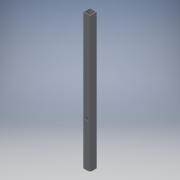
# Autodesk Inventor part: AP 2
Saved by Autodesk Inventor 2016 (Build 200138000, 138)
## iProperties
Created: 2016-02-17
Part Number: AP 2
Material: Generic
Document SubType Name: Modeling
Designer: Admin
Density: 1 g/cm^3
Appearance: Default
Author: Admin
Autodesk Inventor part; units mm, degrees
ref_plane "YZ Plane" through (0, 0, 0) normal (1, 0, 0) x (0, 1, 0)
ref_plane "XZ Plane" through (0, 0, 0) normal (0, 1, 0) x (-1, 0, 0)
ref_plane "XY Plane" through (0, 0, 0) normal (0, 0, 1) x (1, 0, 0)
sketch "Sketch1" plane through (0, 0, 0) normal (0, 1, 0) x (-1, 0, 0)
  line L0 (0, 0) -> (25.4, 0)
  line L1 (25.4, 0) -> (25.4, -25.4)
  line L2 (25.4, -25.4) -> (0, -25.4)
  line L3 (0, -25.4) -> (0, 0)
  line L4 (23.8125, -23.8125) -> (23.8125, -1.5875)
  line L5 (23.8125, -1.5875) -> (1.5875, -1.5875)
  line L6 (1.5875, -1.5875) -> (1.5875, -23.8125)
  line L7 (1.5875, -23.8125) -> (23.8125, -23.8125)
  dimension "d0" = 25.4
  dimension "d1" = 25.4
  dimension "d2" = 1.5875
  constraints: 16 end point, 4 parallel, 2 perpendicular, 1 horizontal, 3 other
  measures "d0" distance of L1.end L2.end
  measures "d1" distance of L0.end L1.end
  measures "d2" distance between parallel lines of L1 L4
extrude "Extrusion1" add sketch "Sketch1" along normal blind 508
sketch "Sketch3" plane through (-25.4, 0, 0) normal (0, 0, 1) x (1, 0, 0)
  point P0 (25.4, 0)
sketch "Sketch4" plane through (-25.4, 0, 0) normal (0, 0, 1) x (1, 0, 0)
  circle A0 centre (12.7, 168.402) radius 6.35
  line L0 (25.4, 0) -> (0, 0) projected
  dimension "d8" = 12.7
  dimension "d9" = 168.402
  constraints: 1 centre point
  measures "d8" diameter of A0
  measures "d9" distance from line of L0 A0.centre
extrude "Extrusion3" cut sketch "Sketch4" against normal blind 25.4
sketch "Sketch5" plane through (-25.4, 0, 0) normal (0, 0, 1) x (1, 0, 0)
  circle A0 centre (12.7, 168.656) radius 6.35
  line L0 (25.4, 0) -> (0, 0) projected
  dimension "d12" = 12.7
  dimension "d15" = 168.656
  constraints: 1 centre point
  measures "d12" diameter of A0
  measures "d15" distance from line of L0 A0.centre
extrude "Extrusion4" cut sketch "Sketch5" against normal blind 25.4
sketch "Sketch6" plane through (0, 0, -25.4) normal (0, 0, -1) x (-1, 0, 0)
  circle A0 centre (10.1854, 83.82) radius 6.35
  line L0 (25.4, 0) -> (0, 0) projected
  line L1 (0, 0) -> (0, 508) projected
  dimension "d16" = 12.7
  dimension "d17" = 83.82
  dimension "d18" = 10.1854
  constraints: 1 centre point
  measures "d16" diameter of A0
  measures "d17" distance from line of L0 A0.centre
  measures "d18" distance from line of L1 A0.centre
extrude "Extrusion5" cut sketch "Sketch6" against normal blind 25.4
sketch "Sketch7" plane through (0, 0, 0) normal (0, -1, 0) x (1, 0, 0)
  line L0 (0, 0) -> (-25.4, 0)
  line L1 (-25.4, 0) -> (-25.4, -25.4)
  line L2 (-25.4, -25.4) -> (0, -25.4)
  line L3 (0, -25.4) -> (0, 0)
  line L4 (-1.5875, -23.8125) -> (-23.8125, -23.8125) projected
  line L5 (-23.8125, -1.5875) -> (-1.5875, -1.5875) projected
  line L6 (-23.8125, -23.8125) -> (-1.5875, -23.8125)
  line L7 (-1.5875, -23.8125) -> (-1.5875, -1.5875)
  line L8 (-1.5875, -1.5875) -> (-23.8125, -1.5875)
  line L9 (-23.8125, -1.5875) -> (-23.8125, -23.8125)
  constraints: 16 end point, 4 parallel, 2 horizontal, 2 perpendicular
extrude "Extrusion6" add sketch "Sketch7" along normal blind 25.4
sketch "Sketch8" plane through (-25.4, 508, 0) normal (0, 0, 1) x (1, 0, 0)
  circle A0 centre (13.081, -508) radius 6.35
  line L0 (25.4, -533.4) -> (25.4, 0) projected
  point P0 (25.4, -508)
  dimension "d23" = 12.7
  dimension "d24" = 12.319
  constraints: 1 centre point
  measures "d23" diameter of A0
  measures "d24" distance from line of L0 A0.centre
extrude "Extrusion7" cut sketch "Sketch8" against normal blind 25.4
body "Solid1"
